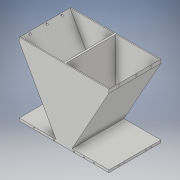
# Autodesk Inventor part: new container
Saved by Autodesk Inventor 2019 (Build 230136000, 136)
## iProperties
Created: 2020-02-28
Part Number: new container
Material: Generic
Document SubType Name: Modeling
Designer: KiranM
Density: 1 g/cm^3
Appearance: Default
Author: KiranM
Autodesk Inventor part; units mm, degrees
ref_plane "YZ Plane" through (0, 0, 0) normal (1, 0, 0) x (0, 1, 0)
ref_plane "XZ Plane" through (0, 0, 0) normal (0, 1, 0) x (-1, 0, 0)
ref_plane "XY Plane" through (0, 0, 0) normal (0, 0, 1) x (1, 0, 0)
sketch "Sketch1" plane through (0, 0, 0) normal (0, 0, 1) x (1, 0, 0)
  line L0 (0, 0) -> (0, 350)
  line L1 (0, 350) -> (450, 350)
  line L2 (450, 350) -> (450, 0)
  line L3 (450, 0) -> (0, 0)
  line L4 (0, 0) -> (225, 0)
  line L5 (225, 350) -> (220, 350)
  line L6 (225, 350) -> (220, 350)
  line L7 (220, 350) -> (230, 350)
  line L8 (230, 350) -> (230, 0)
  line L9 (220, 350) -> (220, 0)
  line L10 (220, 0) -> (195, 0)
  line L11 (230, 0) -> (255, 0)
  line L12 (255, 0) -> (450, 350)
  line L13 (195, 0) -> (0, 350)
  line L14 (255, 0) -> (265, 0)
  line L15 (265, 0) -> (450, 332.0513)
  line L16 (195, 0) -> (185, 0)
  line L17 (185, 0) -> (0, 332.0513)
  line L18 (0, 332.0513) -> (0, 350)
  line L19 (450, 332.0513) -> (450, 350)
  constraints: 40 end point, 9 point on line, 5 perpendicular, 2 collinear, 2 midpoint, 2 parallel, 1 horizontal, 1 vertical
extrude "Extrusion1" add sketch "Sketch1" along normal blind 250 contours L0 L13 L3 L17 | L1 L8 L3 L9 | L2 L15 L3 L12
sketch "Sketch2" plane through (0, 0, 250) normal (0, 0, 1) x (1, 0, 0)
  line L0 (0, 350) -> (0, 332.0513) projected
  line L1 (450, 332.0513) -> (450, 350) projected
  line L2 (0, 350) -> (450, 350)
  line L3 (450, 350) -> (450, 332.0513)
  line L4 (255, 0) -> (265, 0) projected
  line L5 (450, 332.0513) -> (265, 0)
  line L6 (185, 0) -> (195, 0) projected
  line L7 (265, 0) -> (185, 0)
  line L8 (185, 0) -> (0, 332.0513)
  line L9 (0, 332.0513) -> (0, 350)
  point P0 (0, 0)
  constraints: 12 end point, 3 collinear, 1 horizontal
extrude "Extrusion2" add sketch "Sketch2" along normal blind 5
sketch "Sketch3" plane through (0, 0, 0) normal (0, 0, -1) x (-1, 0, 0)
  line L0 (-450, 332.0513) -> (-450, 350) projected
  line L1 (-195, 0) -> (0, 350) projected
  line L2 (-450, 350) -> (0, 350)
  line L3 (0, 350) -> (0, 332.0513) projected
  line L4 (0, 350) -> (0, 332.0513)
  line L5 (0, 332.0513) -> (-185, 0) projected
  line L6 (0, 332.0513) -> (-185, 0)
  line L7 (-185, 0) -> (-265, 0)
  line L8 (-265, 0) -> (-450, 332.0513) projected
  line L9 (-265, 0) -> (-450, 332.0513)
  line L10 (-450, 332.0513) -> (-450, 350)
  point P0 (0, 0)
  constraints: 12 end point, 2 collinear, 2 parallel, 1 horizontal, 1 perpendicular
extrude "Extrusion3" add sketch "Sketch3" along normal blind 5
fillet "Fillet1" radius 2 1 edges at (255, 0, 125)
fillet "Fillet2" radius 2 1 edges at (230, 0, 125)
fillet "Fillet3" radius 2 1 edges at (220, 0, 125)
fillet "Fillet4" radius 2 1 edges at (195, 0, 125)
sketch "Sketch4" plane through (0, 332.0513, 255) normal (-1, 0, 0) x (0, 0, 1)
  line L0 (-255, 17.9487) -> (-260, 17.9487) projected
  line L1 (-260, 17.9487) -> (-260, 8.9744)
  line L2 (-260, 17.9487) -> (-260, 0) projected
  line L3 (-1.0875, 8.9744) -> (-260, 8.9744)
  line L4 (-5, 17.9487) -> (-5, -330.0513) projected
  line L5 (-260, 8.9744) -> (-135, 8.9744)
  circle A0 centre (-135, 8.9744) radius 5
  point P0 (-255, -332.0513)
  dimension "d20" = 125
  dimension "d21" = 10
  constraints: 6 end point, 1 centre point, 1 coincident, 1 midpoint, 1 perpendicular, 1 point on line
  measures "d20" distance of L1.end L5.end
  measures "d21" diameter of A0
extrude "Extrusion4" cut sketch "Sketch4" against normal blind 10
sketch "Sketch5" plane through (450, 332.0513, 255) normal (1, 0, 0) x (0, 0, -1)
  circle A0 centre (135, 8.9744) radius 5 projected
  point P0 (255, -332.0513)
extrude "Extrusion5" cut sketch "Sketch5" against normal blind 10
sketch "Sketch6" plane through (0, 332.0513, 255) normal (-1, 0, 0) x (0, 0, 1)
  circle A0 centre (-135, 8.9744) radius 5 projected
  circle A1 centre (-210, 8.9744) radius 5
  circle A2 centre (-50.1609, 8.9744) radius 5
  point P0 (-255, -332.0513)
  constraints: 2 centre point
extrude "Extrusion6" cut sketch "Sketch6" against normal blind 10 contours A1 | A2
sketch "Sketch7" plane through (450, 332.0513, 255) normal (1, 0, 0) x (0, 0, -1)
  line L0 (5, 17.9487) -> (0, 17.9487) projected
  line L1 (5, 17.9487) -> (5, 8.9487)
  line L2 (5, 17.9487) -> (5, -329.0779) projected
  circle A0 centre (50.1609, 8.9744) radius 5 projected
  line L3 (5, 8.9487) -> (50.1609, 8.9744)
  circle A1 centre (210, 8.9744) radius 5 projected
  circle A2 centre (210, 8.9744) radius 5
  point P0 (255, -332.0513)
  dimension "d40" = 9
  constraints: 4 end point, 1 centre point, 1 coincident, 1 point on line
  measures "d40" distance of L0.start L1.end
extrude "Extrusion7" cut sketch "Sketch7" against normal blind 10 contours A1
sketch "Sketch8" plane through (450, 332.0513, 255) normal (1, 0, 0) x (0, 0, -1)
  circle A0 centre (50.1609, 8.9744) radius 5 projected
  circle A1 centre (50.1609, 8.9744) radius 5
  point P0 (255, -332.0513)
  constraints: 1 centre point, 1 coincident
extrude "Extrusion8" cut sketch "Sketch8" against normal blind 10
sketch "Sketch9" plane through (185, 0, 255) normal (0, -1, 0) x (1, 0, 0)
  line L0 (-185, -260) -> (-185, 0) projected
  line L1 (265, -260) -> (-185, -260)
  line L2 (-185, -260) -> (-185, 0)
  line L3 (-185, 0) -> (265, 0)
  line L4 (265, 0) -> (265, -260)
  point P0 (-185, -255)
  constraints: 8 end point, 2 parallel, 1 horizontal, 1 perpendicular
extrude "Extrusion9" add sketch "Sketch9" along normal blind 12
sketch "Sketch10" plane through (185, -12, 255) normal (0, -1, 0) x (1, 0, 0)
  line L0 (35, -5) -> (35, -255) projected
  line L1 (14.5122, -257.9685) -> (35, -257.9685)
  line L2 (35, -257.9685) -> (35, -5)
  line L3 (35, -5) -> (14.5122, -5)
  line L4 (14.5122, -5) -> (14.5122, -257.9685)
  point P0 (-185, -255)
  constraints: 8 end point, 2 parallel, 1 horizontal, 1 perpendicular
extrude "Extrusion10" cut sketch "Sketch10" against normal blind 12
sketch "Sketch11" plane through (185, 0, 255) normal (0, 1, 0) x (1, 0, 0)
  line L0 (73.4037, 255) -> (43, 255) projected
  line L1 (45.375, 255) -> (71.2984, 255)
  line L2 (71.2984, 255) -> (71.2984, 5.0453)
  line L3 (71.2984, 5.0453) -> (45.375, 5.0453)
  line L4 (45.375, 5.0453) -> (45.375, 255)
  point P0 (-185, 255)
  constraints: 8 end point, 2 parallel, 1 horizontal, 1 perpendicular, 1 point on line
extrude "Extrusion11" cut sketch "Sketch11" against normal blind 12
sketch "Sketch12" plane through (450, 0, 255) normal (1, 0, 0) x (0, 0, -1)
  circle A0 centre (50.1609, -6.6697) radius 2.5
  circle A1 centre (211.0368, -6.6697) radius 2.5
  point P0 (255, 0)
  constraints: 2 centre point
extrude "Extrusion12" cut sketch "Sketch12" against normal blind 10 contours A1
sketch "Sketch13" plane through (450, 0, 255) normal (1, 0, 0) x (0, 0, -1)
  circle A0 centre (49.8818, -6) radius 2.5
  point P0 (255, 0)
  constraints: 1 centre point
extrude "Extrusion13" cut sketch "Sketch13" against normal blind 25
sketch "Sketch14" plane through (0, 0, -5) normal (-1, 0, 0) x (0, 0, 1)
  circle A0 centre (48.9632, -6.6697) radius 2.5 projected
  point P0 (5, 0)
extrude "Extrusion14" cut sketch "Sketch14" against normal blind 25
sketch "Sketch15" plane through (0, 0, -5) normal (-1, 0, 0) x (0, 0, 1)
  circle A0 centre (209.8391, 341.0256) radius 5 projected
  circle A1 centre (210.1182, -6) radius 2.5 projected
  circle A2 centre (210.1182, -6) radius 2.5
  point P0 (5, 0)
  constraints: 1 centre point, 1 coincident
extrude "Extrusion15" cut sketch "Sketch15" against normal blind 25 contours A1
sketch "Sketch16" plane through (0, 0, 255) normal (0, 0, 1) x (1, 0, 0)
  circle A0 centre (175, -8) radius 2.5
  circle A1 centre (325, -8) radius 2.5
  point P0 (0, 0)
  constraints: 2 centre point
extrude "Extrusion16" cut sketch "Sketch16" against normal blind 25
sketch "Sketch17" plane through (0, 0, -5) normal (0, 0, -1) x (-1, 0, 0)
  line L0 (0, 0) -> (0, -8)
  circle A0 centre (-175, -8) radius 2.5 projected
  circle A1 centre (-325, -8) radius 2.5
  constraints: 2 end point, 1 centre point, 1 vertical
extrude "Extrusion17" cut sketch "Sketch17" against normal blind 25
sketch "Sketch18" plane through (0, 0, 255) normal (0, 0, 1) x (1, 0, 0)
  circle A0 centre (275.1205, -8.1253) radius 2.5
  point P0 (0, 0)
  constraints: 1 centre point
extrude "Extrusion18" cut sketch "Sketch18" against normal blind 25
sketch "Sketch19" plane through (0, 0, -5) normal (0, 0, -1) x (-1, 0, 0)
  line L0 (-175.0524, -7.9196) -> (-275.0524, -7.9196)
  circle A0 centre (-275.0524, -7.9196) radius 2.5
  point P0 (0, 0)
  dimension "d85" = 100
  dimension "d86" = 5
  constraints: 2 end point, 1 centre point, 1 coincident, 1 horizontal
  measures "d85" distance of L0.start L0.end
  measures "d86" diameter of A0
extrude "Extrusion19" cut sketch "Sketch19" against normal blind 25
sketch "Sketch20" plane through (0, 0, 255) normal (0, 0, 1) x (1, 0, 0)
  line L0 (0, 0) -> (0, -4.6382)
  circle A0 centre (75, -4.6382) radius 2.5
  line L1 (450, 0) -> (265, 0) projected
  line L2 (450, 0) -> (450, -6)
  line L3 (450, 0) -> (450, -12) projected
  circle A1 centre (375, -6) radius 2.5
  constraints: 4 end point, 2 centre point, 1 midpoint, 1 vertical
extrude "Extrusion20" cut sketch "Sketch20" against normal blind 25
sketch "Sketch21" plane through (450, 0, 255) normal (1, 0, 0) x (0, 0, -1)
  circle A0 centre (75, -5.6253) radius 2.5
  circle A1 centre (185, -6) radius 2.5
  point P0 (255, 0)
  constraints: 2 centre point
extrude "Extrusion21" cut sketch "Sketch21" against normal blind 25
sketch "Sketch22" plane through (0, 0, -5) normal (-1, 0, 0) x (0, 0, 1)
  circle A0 centre (75, -6) radius 2.5
  line L0 (260, 0) -> (260, -12) projected
  circle A1 centre (185, -5.9997) radius 2.5
  point P0 (5, 0)
  constraints: 2 centre point
extrude "Extrusion22" cut sketch "Sketch22" against normal blind 25
body "Solid1"
